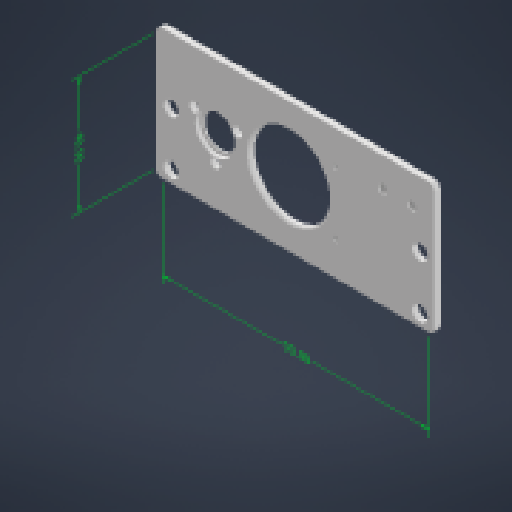
# Autodesk Inventor part: płyta silnika
Saved by Autodesk Inventor 2026.1 (Build 301233020, 233B)
## iProperties
Created: 2026-02-25
Part Number: płyta silnika
Material: Generic
Document SubType Name: Modeling
Designer: Jan
Density: 1 g/cm^3
Appearance: Default
Author: Jan
Autodesk Inventor part; units mm, degrees
ref_plane "YZ Plane" through (0, 0, 0) normal (1, 0, 0) x (0, 1, 0)
ref_plane "XZ Plane" through (0, 0, 0) normal (0, 1, 0) x (-1, 0, 0)
ref_plane "XY Plane" through (0, 0, 0) normal (0, 0, 1) x (1, 0, 0)
sketch "Sketch1" plane through (0, 0, 0) normal (0, 1, 0) x (-1, 0, 0)
  line L0 (0, 0) -> (-40, 0)
  line L1 (-40, 0) -> (-40, -2)
  line L2 (-40, -2) -> (0, -2)
  line L3 (0, -2) -> (0, 0)
  dimension "d0" = 40
  dimension "d1" = 2
  constraints: 8 end point, 2 parallel, 1 horizontal, 1 perpendicular
  measures "d0" distance of L2.end L1.end
  measures "d1" distance of L1.end L0.end
extrude "Extrusion1" add sketch "Sketch1" along normal blind 44
sketch "Sketch2" plane through (0, 0, 0) normal (0, 0, 1) x (1, 0, 0)
  line L0 (40, 44) -> (0, 44) construction
  line L1 (0, 44) -> (40, 0) construction
  line L2 (40, 44) -> (0, 0) construction
  circle A0 centre (20, 22) radius 6.75
  dimension "d4" = 13.5
  constraints: 4 end point, 1 centre point, 1 midpoint
  measures "d4" diameter of A0
extrude "Extrusion2" cut sketch "Sketch2" against normal blind 40
sketch "Sketch3" plane through (40, 0, -2) normal (0, 0, -1) x (-1, 0, 0)
  circle A0 centre (20, 22) radius 6.75 construction
  circle A1 centre (20, 22) radius 8.5 construction
  circle A2 centre (12.6388, 26.25) radius 1.1 construction
  circle A3 centre (27.3612, 26.25) radius 1.1 construction
  line L0 (20, 22) -> (27.3612, 26.25) construction
  line L1 (20, 22) -> (12.6388, 26.25) construction
  circle A4 centre (20, 13.5) radius 1.1 construction
  line L2 (20, 22) -> (20, 13.5) construction
  line L3 (40, 0) -> (40, 44) construction
  dimension "d7" = 17
  dimension "d9" = 2.2
  dimension "d10" = 2.2
  dimension "d22" = 2.2
  dimension "d25" = 120
  dimension "d26" = 120
  constraints: 6 end point, 4 centre point, 3 point on circle, 2 coincident, 1 parallel
  measures "d7" diameter of A1
  measures "d9" diameter of A2
  measures "d10" diameter of A3
  measures "d22" diameter of A4
  measures "d25" angle of L0 L2
  measures "d26" angle of L1 L2
hole "Hole1" at (20, 13.5, -2) at (12.6388, 26.25, -2) at (27.3612, 26.25, -2) direction (0, 0, 1) diameter 3.1 depth 8.8 tip angle 118 clearance for "Countersunk Flat Head Screw ISO 2009/7046" size "M3" standard "ISO"
sketch "Sketch4" plane through (40, 0, 0) normal (1, 0, 0) x (0, 0, -1)
  line L0 (0, 44) -> (2, 44) projected
  line L1 (0, 0) -> (2, 0)
  line L2 (2, 0) -> (2, 44)
  line L3 (2, 44) -> (0, 44)
  line L4 (0, 44) -> (0, 0)
  constraints: 8 end point, 2 parallel, 1 horizontal, 1 perpendicular
extrude "Extrusion3" add sketch "Sketch4" along normal blind 20
sketch "Sketch5" plane through (0, 0, -2) normal (0, 0, -1) x (-1, 0, 0)
  circle A0 centre (-44.75, 22) radius 13.2
  line L0 (0, 0) -> (-60, 0) projected
  line L1 (-60, 0) -> (-60.0955, 41.9998)
  line L2 (0, 0) -> (0, 44) projected
  dimension "d27" = 26.4
  dimension "d28" = 22
  dimension "d29" = 15.3
  dimension "d45" = 44.75
  constraints: 2 end point, 1 centre point
  measures "d27" diameter of A0
  measures "d28" distance from line of A0.centre L0
  measures "d29" distance from line of L1 A0.centre
  measures "d45" distance from line of A0.centre L2
extrude "Extrusion4" cut sketch "Sketch5" against normal through all
sketch "Sketch6" plane through (60, 0, 0) normal (1, 0, 0) x (0, 0, -1)
  line L0 (0, 0) -> (0, 44) projected
  line L1 (2, 0) -> (0, 0) projected
  line L2 (0, 44) -> (2, 44)
  line L3 (2, 44) -> (2, 0)
  line L4 (2, 0) -> (0, 0)
  line L5 (0, 0) -> (0, 44)
  constraints: 8 end point, 2 parallel, 1 horizontal, 1 perpendicular
extrude "Extrusion5" add sketch "Sketch6" along normal blind 34
fillet "Fillet1" radius 2 4 edges at (0, 44, -1) (0, 0, -1) (94, 44, -1) (94, 0, -1)
sketch "Sketch7" plane through (2, 0, 0) normal (0, 0, 1) x (1, 0, 0)
  circle A0 centre (87, 22) radius 2.5
  circle A1 centre (3, 22) radius 2.5
  line L0 (0, 44) -> (90, 44) projected
  line L1 (92, 42) -> (92, 2) projected
  line L2 (0, 0) -> (90, 0) projected
  line L3 (-2, 2) -> (-2, 42) projected
  circle A2 centre (87, 4) radius 2.5
  circle A3 centre (3, 4) radius 2.5
  point P0 (-2, 0)
  dimension "d53" = 5
  dimension "d54" = 5
  dimension "d55" = 22
  dimension "d56" = 5
  dimension "d57" = 22
  dimension "d58" = 5
  dimension "d69" = 44
  dimension "d73" = 5
  dimension "d74" = 18
  dimension "d75" = 5
  constraints: 4 centre point
  measures "d53" diameter of A0
  measures "d54" diameter of A1
  measures "d55" distance from line of L0 A0.centre
  measures "d56" distance from line of L1 A0.centre
  measures "d57" distance from line of L2 A1.centre
  measures "d58" distance from line of L3 A1.centre
  measures "d69" distance between parallel lines of L0 L2
  measures "d73" diameter of A2
  measures "d74" distance of A2.centre A0.centre
  measures "d75" diameter of A3
hole "Hole2" at (5, 22, 0) at (89, 22, 0) at (89, 4, 0) at (5, 4, 0) direction (0, 0, -1) diameter 5 depth 14.2 tip angle 118
chamfer "Chamfer1" distance 0.3 angle 45 2 edges at (5, 24.5, -2) (89, 24.5, -2)
sketch "Sketch8" plane through (92, 0, -2) normal (0, 0, -1) x (-1, 0, 0)
  circle A0 centre (72, 22) radius 6.75 projected
  circle A1 centre (72, 22) radius 6.75
  circle A2 centre (72, 22) radius 5.5
  point P0 (92, 0)
  dimension "d70" = 11
  constraints: 3 coincident, 2 centre point, 1 concentric
  measures "d70" diameter of A2
extrude "Extrusion6" add sketch "Sketch8" against normal blind 0.6
sketch "Sketch9" plane through (2, 0, 0) normal (0, 0, 1) x (1, 0, 0)
  circle A0 centre (58.5, 32.48) radius 1
  circle A1 centre (58.5, 11.52) radius 1
  line L0 (0, 44) -> (90, 44) projected
  line L1 (0, 0) -> (90, 0) projected
  line L2 (92, 42) -> (92, 2) projected
  point P0 (-2, 0)
  dimension "d76" = 2
  dimension "d77" = 2
  dimension "d78" = 20.96
  dimension "d79" = 44
  dimension "d80" = 11.52
  dimension "d81" = 33.5
  constraints: 2 centre point, 1 vertical alignment
  measures "d76" diameter of A0
  measures "d77" diameter of A1
  measures "d78" distance of A0.centre A1.centre
  measures "d79" distance between parallel lines of L0 L1
  measures "d80" distance from line of L1 A1.centre
  measures "d81" distance from line of A1.centre L2
hole "Hole3" at (60.5, 11.52, 0) at (60.5, 32.48, 0) direction (0, 0, -1) diameter 1.567 depth 6.3 tip angle 118 thread size "M2x0.4" class "6H" standard "ISO Metric profile"
chamfer "Chamfer2" distance 0.5 angle 45 1 edges at (57.95, 22, 0)
chamfer "Chamfer3" distance 0.2 angle 45 2 edges at (60.5, 12.3035, 0) (60.5, 33.2635, 0)
sketch "Sketch10" plane through (2, 0, 0) normal (0, 0, 1) x (1, 0, 0)
  circle A0 centre (84.365, 34) radius 1
  circle A1 centre (74.365, 34) radius 1
  line L0 (0, 44) -> (90, 44) projected
  line L1 (92, 42) -> (92, 2) projected
  point P0 (-2, 0)
  dimension "d95" = 2
  dimension "d96" = 2
  dimension "d97" = 10
  dimension "d98" = 10
  dimension "d99" = 7.635
  constraints: 2 centre point, 1 horizontal alignment
  measures "d95" diameter of A0
  measures "d96" diameter of A1
  measures "d97" distance of A1.centre A0.centre
  measures "d98" distance from line of A0.centre L0
  measures "d99" distance from line of A0.centre L1
hole "Hole4" at (86.365, 34, 0) at (76.365, 34, 0) direction (0, 0, -1) diameter 2.459 depth 8.8 tip angle 118 thread size "M3x0.5" class "6H" standard "ISO Metric profile"
chamfer "Chamfer4" distance 0.3 angle 45 2 edges at (86.365, 35.2295, 0) (76.365, 35.2295, 0)
equation "\"d55\" = 0.5 * d69"
equation "\"d57\" = 0.5 * d69"
equation "\"d80\" = -0.5 * d78 + 0.5 * d79"
body "Solid1"
